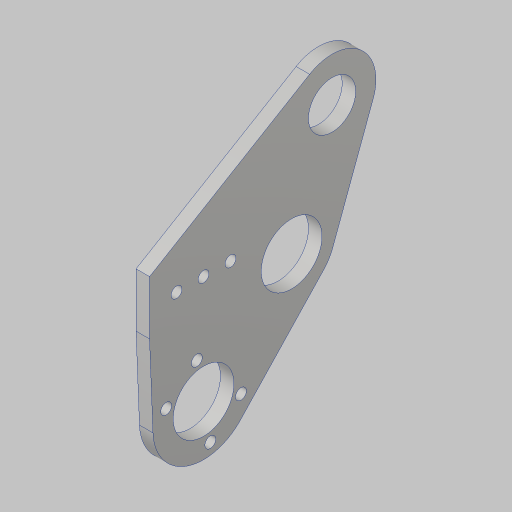
# Autodesk Inventor part: GP5-011
Saved by Autodesk Inventor 2023.5 (Build 275446000, 446)
## iProperties
Created: 2025-02-03
Part Number: GP5-011
Material: Aluminum 6061
Document SubType Name: Modeling
Designer: slick
Density: 2.7 g/cm^3
Appearance: Aluminum - Flat
Author: slick
Autodesk Inventor part; units mm, degrees
ref_plane "YZ Plane" through (0, 0, 0) normal (1, 0, 0) x (0, 1, 0)
ref_plane "XZ Plane" through (0, 0, 0) normal (0, 1, 0) x (-1, 0, 0)
ref_plane "XY Plane" through (0, 0, 0) normal (0, 0, 1) x (1, 0, 0)
sketch "Sketch1" plane through (0, 0, 0) normal (1, 0, 0) x (0, 1, 0)
  line L0 (-12.7, 25.4) -> (12.7, 25.4) construction
  line L1 (12.7, 25.4) -> (12.7, -25.4) construction
  line L2 (12.7, -25.4) -> (-12.7, -25.4) construction
  line L3 (-12.7, -25.4) -> (-12.7, 25.4) construction
  line L4 (-12.7, 25.4) -> (12.7, -25.4) construction
  line L5 (12.7, 25.4) -> (-12.7, -25.4) construction
  circle A0 centre (-50.8, 0) radius 14.2875
  circle A1 centre (-127, -49.5046) radius 38.1 construction
  circle A2 centre (-50.8, 0) radius 23.8125 construction
  circle A3 centre (76.2, -50.8) radius 5.9531 construction
  circle A4 centre (39.7562, -60.4629) radius 31.75 construction
  circle A5 centre (76.2, -50.8) radius 17.4625 construction
  circle A6 centre (76.2, -50.8) radius 22.098 construction
  line L6 (12.7, -25.4) -> (215.9, -25.4) construction
  line L7 (215.9, -25.4) -> (215.9, 25.4) construction
  line L8 (215.9, 25.4) -> (12.7, 25.4) construction
  line L9 (-51.7788, 23.7924) -> (-12.7, 25.4)
  line L10 (-12.7, 25.4) -> (12.7, 25.4)
  line L11 (12.7, 25.4) -> (57.4935, -49.9134)
  arc A7 (-51.7788, 23.7924) -> (-67.1218, -17.3388) centre (-50.8, 0) ccw
  circle A8 centre (39.7562, -60.4629) radius 12.7 construction
  circle A9 centre (-11.4274, -41.4237) radius 41.91 construction
  circle A10 centre (-11.4274, -41.4237) radius 19.05 construction
  circle A11 centre (-50.8, 0) radius 38.1 construction
  circle A12 centre (39.7562, -60.4629) radius 11.1125
  circle A13 centre (-11.4274, -41.4237) radius 14.2875
  circle A14 centre (39.7562, -60.4629) radius 20.6375 construction
  circle A15 centre (-11.4274, -41.4237) radius 20.6375 construction
  line L12 (32.5611, -79.8056) -> (-18.6225, -60.7663)
  line L13 (-25.573, -56.4506) -> (-67.1218, -17.3388)
  arc A16 (32.5611, -79.8056) -> (57.4935, -49.9134) centre (39.7562, -60.4629) ccw
  arc A17 (-25.573, -56.4506) -> (-18.6225, -60.7663) centre (-11.4274, -41.4237) ccw
  circle A18 centre (50.8, -31.75) radius 6.35 construction
  line L14 (-56.5816, -17.5873) -> (-69.039, -3.175) construction
  line L15 (-69.039, -3.175) -> (-45.0184, 17.5873) construction
  line L16 (-45.0184, 17.5873) -> (-32.561, 3.175) construction
  line L17 (-32.561, 3.175) -> (-56.5816, -17.5873) construction
  line L18 (-56.5816, -17.5873) -> (-45.0184, 17.5873) construction
  line L19 (-69.039, -3.175) -> (-32.561, 3.175) construction
  point P0 (0, 0)
  point P1 (0, -12.7)
  point P2 (0, 0)
  point P3 (0, 12.7)
  point P4 (81.0318, -72.3633)
  point P5 (-39.5444, 23.7687)
  point P6 (76.2, -50.8)
  point P7 (76.2, -68.2625)
  point P8 (91.323, -59.5312)
  point P9 (91.323, -42.0687)
  point P10 (76.2, -33.3375)
  point P11 (61.077, -42.0687)
  point P12 (61.077, -59.5312)
  dimension "d20" = 34.925
  dimension "d21" = 44.196
  dimension "d0" = 25.4
  dimension "d1" = 50.8
  dimension "d2" = 28.575
  dimension "d3" = 50.8
  dimension "d4" = 76.2
  dimension "d5" = 127
  dimension "d6" = 49.5046
  dimension "d11" = 12.7
  dimension "d12" = 12.7
  dimension "d13" = 9.525
  dimension "d18" = 11.9062
  dimension "d19" = 63.5
  dimension "d22" = 203.2
  dimension "d23" = 25.4
  dimension "d24" = 63.5
  dimension "d31" = 360
  dimension "d40" = 25.4
  dimension "d41" = 83.82
  dimension "d42" = 38.1
  dimension "d43" = 76.2
  dimension "d44" = 36.4438
  dimension "d46" = 6.35
  dimension "d48" = 12.7
  dimension "d49" = 25.4
  dimension "d50" = 22.225
  dimension "d51" = 31.75
  dimension "d52" = 19.05
  dimension "d54" = 3.175
  constraints: 40 end point, 17 centre point, 16 coincident, 12 point on circle, 10 tangent, 5 vertical alignment, 4 parallel, 4 perpendicular, 3 equal radius, 3 midpoint, 2 horizontal, 1 horizontal alignment, 12 other
  measures "d0" distance of L1.end L2.end
  measures "d1" distance of L0.end L1.end
  measures "d2" diameter of A0
  measures "d3" distance of A0.centre point (0, 0)
  measures "d4" diameter of A1
  measures "d5" horizontal distance of A1.centre point (0, 0)
  measures "d6" vertical distance of A1.centre point (0, 0)
  measures "d11" distance of point (0, -12.7) point (0, 0)
  measures "d12" distance of point (0, 0) point (0, 12.7)
  measures "d13" radial gap between concentric circles of A0 A2
  measures "d18" diameter of A3
  measures "d19" diameter of A4
  measures "d22" distance between parallel lines of L1 L7
  measures "d23" distance from line of L6 point (76.2, -50.8)
  measures "d24" horizontal distance of L1.end A3.centre
  measures "d40" diameter of A8
  measures "d41" diameter of A9
  measures "d42" diameter of A10
  measures "d43" diameter of A11
  measures "d44" horizontal distance of A3.centre A4.centre
  measures "d46" radial gap between concentric circles of A13 A15
  measures "d48" diameter of A18
  measures "d49" horizontal distance of A18.centre A3.centre
  measures "d50" diameter of A12
  measures "d51" distance of L14.end L15.end
  measures "d52" distance of L14.end L14.start
  measures "d54" vertical distance of L16.end point (0, 0)
extrude "Extrusion1" add sketch "Sketch1" along normal blind 6.35
hole "Hole1" at (0, 0, -12.7) at (0, 0, 0) at (0, 0, 12.7) direction (1, 0, 0) diameter 5.1054 end through all clearance for "Flat Head Machine Screw (82)" size "#10" standard "Ansi Unified Screw Threads"
hole "Hole2" at (0, -69.039, -3.175) at (0, -56.5816, -17.5873) at (0, -32.561, 3.175) at (0, -45.0184, 17.5873) direction (1, 0, 0) diameter 5.1054 end through all clearance for "Flat Head Machine Screw (82)" size "#10" standard "Ansi Unified Screw Threads"
equation "\"d12\" = d11"
body "Solid1"
